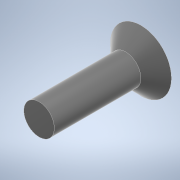
# Autodesk Inventor part: DIN 912 M3 10 mm
Saved by Autodesk Inventor 2022 (Build 260153000, 153)
## iProperties
Created: 2021-10-06
Part Number: DIN 912 M3 10 mm
Material: Generic
Document SubType Name: Modeling
Designer: Administrator
Density: 1 g/cm^3
Appearance: Smooth - Black
Title: DIN 912 M3 10 mm
Author: Administrator
Autodesk Inventor part; units mm, degrees
ref_plane "YZ Plane" through (0, 0, 0) normal (1, 0, 0) x (0, 1, 0)
ref_plane "XZ Plane" through (0, 0, 0) normal (0, 1, 0) x (-1, 0, 0)
ref_plane "XY Plane" through (0, 0, 0) normal (0, 0, 1) x (1, 0, 0)
sketch "Sketch1" plane through (0, 0, 0) normal (1, 0, 0) x (0, 1, 0)
  line L0 (0, 0) -> (0, -10)
  line L1 (0, -10) -> (3, -10)
  line L2 (3, -10) -> (1.5, -8.5)
  line L3 (1.5, -8.5) -> (1.5, 0)
  line L4 (1.5, 0) -> (0, 0)
  dimension "d0" = 6
  dimension "d1" = 10
  dimension "d2" = 45
  dimension "d3" = 3
  constraints: 10 end point, 2 horizontal, 1 perpendicular, 1 vertical
  measures "d0" diameter of L1.end L0
  measures "d1" distance between parallel lines of L4 L1
  measures "d2" angle of L1 L2
  measures "d3" diameter of L3 L0
revolve "Revolution1" add sketch "Sketch1" angle 360 about axis through (0, 0, 0) along (0, 0, -1)
body "Solid2"
